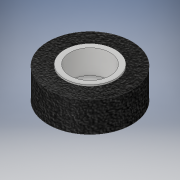
# Autodesk Inventor part: Antriebsrad_V1
Saved by Autodesk Inventor 2017.3 (Build 213257000, 257)
## iProperties
Part Number: Antriebsrad_V1
Material: Generisch
Document SubType Name: Modeling
Designer: Enno-LT
Density: 1 g/cm^3
Appearance: Vorgabe
Author: Enno-LT
Autodesk Inventor part; units mm, degrees
ref_plane "YZ Plane" through (0, 0, 0) normal (1, 0, 0) x (0, 1, 0)
ref_plane "XZ Plane" through (0, 0, 0) normal (0, 1, 0) x (-1, 0, 0)
ref_plane "XY Plane" through (0, 0, 0) normal (0, 0, 1) x (1, 0, 0)
sketch "Skizze2" plane through (0, 0, 0) normal (0, 0, 1) x (1, 0, 0)
  circle A0 centre (0, 0) radius 9.5
  circle A1 centre (0, 0) radius 15.6
  dimension "d2" = 19
  dimension "d3" = 31.2
  constraints: 3 coincident, 2 centre point
  measures "d2" diameter of A0
  measures "d3" diameter of A1
extrude "Extrusion1" add sketch "Skizze2" along normal mid plane 11.2
sketch "Skizze3" plane through (0, 0, 5.6) normal (0, 0, 1) x (1, 0, 0)
  circle A0 centre (0, 0) radius 9.45
  dimension "d6" = 18.9
  constraints: 2 coincident, 1 centre point
  measures "d6" diameter of A0
extrude "Extrusion2" add sketch "Skizze3" along normal blind 0.5 and the other way blind 11.2
fillet "Rundung1" radius 0.5 1 edges at (-9.45, 0, -5.6)
fillet "Rundung2" radius 0.5 1 edges at (-9.5, 0, -5.6)
sketch "Skizze4" plane through (0, 0, 6.1) normal (0, 0, 1) x (1, 0, 0)
  circle A0 centre (0, 0) radius 7.5
  dimension "d13" = 15
  constraints: 1 centre point, 1 coincident
  measures "d13" diameter of A0
extrude "Extrusion3" cut sketch "Skizze4" against normal blind 9
sketch "Skizze6" plane through (0, 0, -5.6) normal (0, 0, -1) x (-1, 0, 0)
  circle A0 centre (0, 0) radius 4.75
  dimension "d23" = 9.5
  constraints: 1 centre point, 1 coincident
  measures "d23" diameter of A0
extrude "Extrusion4" add sketch "Skizze6" along normal blind 5
sketch "Skizze7" plane through (0, 0, -10.6) normal (0, 0, -1) x (-1, 0, 0)
  point P0 (0, 0)
  point P1 (0, 0)
  point P2 (0, 0)
  constraints: 2 coincident
hole "Bohrung2" at (0, 0, -10.6) direction (0, 0, 1) diameter 2.5 end through all
sketch "Skizze8" plane through (0, 0, 0) normal (0, 1, 0) x (-1, 0, 0)
  line L0 (0, 0) -> (0, -22.2603) construction
  line L1 (-4.75, -5.6) -> (-4.75, -10.6) projected
  line L2 (-4.75, -8.1) -> (11.4066, -8.1) construction
  point P0 (0, -8.1)
  constraints: 4 end point, 2 point on line, 1 horizontal, 1 midpoint, 1 vertical
hole "Bohrung3" at (0, 0, -8.1) direction (0, 1, 0) diameter 2 depth 6.75 tip angle 118
thread "Gewinde1" size "M2x0.4" class "6H" standard "ANSI Metric M Profile" full length
